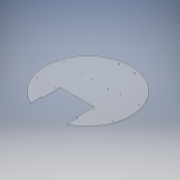
# Autodesk Inventor part: TopPlate
Saved by Autodesk Inventor 2019 (Build 230136000, 136)
## iProperties
Created: 2019-09-28
Part Number: TopPlate
Material: Generic
Document SubType Name: Modeling
Designer: james
Density: 1 g/cm^3
Appearance: Polycarbonate - Clear
Mass: 617.456 g
Surface Area: 2657.72 cm^2
Volume: 617.456 cm^3
Author: james
Autodesk Inventor part; units mm, degrees
ref_plane "YZ Plane" through (0, 0, 0) normal (1, 0, 0) x (0, 1, 0)
ref_plane "XZ Plane" through (0, 0, 0) normal (0, 1, 0) x (-1, 0, 0)
ref_plane "XY Plane" through (0, 0, 0) normal (0, 0, 1) x (1, 0, 0)
sketch "Sketch1" plane through (0, 0, 0) normal (0, 1, 0) x (-1, 0, 0)
  circle A0 centre (0, 0) radius 203.2
  dimension "d0" = 406.4
  constraints: 1 centre point, 1 coincident
  measures "d0" diameter of A0
extrude "Extrusion1" add sketch "Sketch1" along normal blind 4.7625
sketch "Sketch2" plane through (0, 4.7625, 0) normal (0, 1, 0) x (1, 0, 0)
  point P0 (0, 0)
  point P1 (-88.9, 64)
  point P2 (-176.9, 64)
  point P3 (-88.9, -64)
  point P4 (-176.9, -64)
  dimension "d3" = 0
  dimension "d4" = 0
  dimension "d5" = 0
  dimension "d6" = 0
  dimension "d7" = 128
  dimension "d8" = 88
  dimension "d9" = 64
  dimension "d10" = 88.9
  measures "d3" horizontal distance of point (-176.9, -64) point (-176.9, 64)
  measures "d4" horizontal distance of point (-88.9, -64) point (-88.9, 64)
  measures "d5" vertical distance of point (-176.9, -64) point (-88.9, -64)
  measures "d6" vertical distance of point (-176.9, 64) point (-88.9, 64)
  measures "d7" distance of point (-176.9, -64) point (-176.9, 64)
  measures "d8" distance of point (-176.9, -64) point (-88.9, -64)
  measures "d9" vertical distance of point (-88.9, -64) point (0, 0)
  measures "d10" horizontal distance of point (-88.9, 64) point (0, 0)
hole "Hole1" at (-88.9, 4.7625, -64) at (-176.9, 4.7625, -64) at (-88.9, 4.7625, 64) at (-176.9, 4.7625, 64) direction (0, -1, 0) diameter 3.2766 end through all clearance for "Flat Head Machine Screw (82)" size "#4" standard "Ansi Unified Screw Threads"
sketch "Sketch3" plane through (0, 4.7625, 0) normal (0, 1, 0) x (1, 0, 0)
  point P0 (0, 0)
  point P1 (88.9, 64)
  point P2 (176.9, 64)
  point P3 (88.9, -62)
  point P4 (176.9, -62)
  dimension "d18" = 0
  dimension "d19" = 0
  dimension "d20" = 0
  dimension "d21" = 0
  dimension "d22" = 126
  dimension "d23" = 88
  dimension "d24" = 64
  dimension "d25" = 88.9
  measures "d18" horizontal distance of point (176.9, -62) point (176.9, 64)
  measures "d19" vertical distance of point (88.9, 64) point (176.9, 64)
  measures "d20" vertical distance of point (88.9, -62) point (176.9, -62)
  measures "d21" horizontal distance of point (88.9, 64) point (88.9, -62)
  measures "d22" distance of point (176.9, -62) point (176.9, 64)
  measures "d23" distance of point (88.9, -62) point (176.9, -62)
  measures "d24" vertical distance of point (0, 0) point (88.9, 64)
  measures "d25" horizontal distance of point (0, 0) point (88.9, -62)
hole "Hole2" at (88.9, 4.7625, -64) at (176.9, 4.7625, -64) at (88.9, 4.7625, 62) at (176.9, 4.7625, 62) direction (0, -1, 0) diameter 3.2766 end through all clearance for "Flat Head Machine Screw (82)" size "#4" standard "Ansi Unified Screw Threads"
sketch "Sketch4" plane through (0, 4.7625, 0) normal (0, 1, 0) x (1, 0, 0)
  point P0 (0, 0)
  point P1 (-38.1, 184.15)
  point P2 (38.1, 184.15)
  dimension "d33" = 38.1
  dimension "d34" = 0
  dimension "d35" = 76.2
  dimension "d36" = 184.15
  measures "d33" horizontal distance of point (-38.1, 184.15) point (0, 0)
  measures "d34" vertical distance of point (38.1, 184.15) point (-38.1, 184.15)
  measures "d35" distance of point (-38.1, 184.15) point (38.1, 184.15)
  measures "d36" vertical distance of point (0, 0) point (-38.1, 184.15)
hole "Hole3" at (-38.1, 4.7625, -184.15) at (38.1, 4.7625, -184.15) direction (0, -1, 0) diameter 5.1054 end through all clearance for "Flat Head Machine Screw (82)" size "#10" standard "Ansi Unified Screw Threads"
sketch "Sketch5" plane through (0, 4.7625, 0) normal (0, 1, 0) x (1, 0, 0)
  line L0 (-79.375, -50.8) -> (79.375, -50.8)
  line L1 (79.375, -50.8) -> (79.375, -418.3154)
  line L2 (79.375, -418.3154) -> (-79.375, -418.3154)
  line L3 (-79.375, -418.3154) -> (-79.375, -50.8)
  point P0 (0, 0)
  dimension "d44" = 158.75
  dimension "d45" = 79.375
  dimension "d46" = 50.8
  constraints: 8 end point, 2 parallel, 1 horizontal, 1 perpendicular
  measures "d44" distance of L1.end L2.end
  measures "d45" distance from line of L3 point (0, 0)
  measures "d46" distance from line of L0 point (0, 0)
extrude "Extrusion2" cut sketch "Sketch5" against normal blind 25.4
sketch "Sketch6" plane through (0, 4.7625, 0) normal (0, 1, 0) x (1, 0, 0)
  line L0 (-85.725, -133.35) -> (85.725, -133.35)
  line L1 (85.725, -133.35) -> (85.725, -214.7916)
  line L2 (85.725, -214.7916) -> (-85.725, -214.7916)
  line L3 (-85.725, -214.7916) -> (-85.725, -133.35)
  line L4 (-79.375, -50.8) -> (79.375, -50.8) projected
  line L5 (-79.375, -187.0557) -> (-79.375, -50.8) projected
  line L6 (79.375, -50.8) -> (79.375, -187.0557) projected
  point P0 (0, 0)
  dimension "d49" = 82.55
  dimension "d50" = 6.35
  dimension "d51" = 6.35
  constraints: 8 end point, 2 parallel, 1 horizontal, 1 perpendicular
  measures "d49" distance between parallel lines of L0 L4
  measures "d50" distance between parallel lines of L3 L5
  measures "d51" distance between parallel lines of L6 L1
extrude "Extrusion3" cut sketch "Sketch6" against normal blind 25.4 contours L0 L1 L2 L3
sketch "Sketch7" plane through (0, 4.7625, 0) normal (0, 1, 0) x (1, 0, 0)
  circle A0 centre (38.1, 184.15) radius 2.5527 projected
  circle A1 centre (-38.1, 184.15) radius 2.5527 projected
  point P0 (0, 0)
  point P1 (-38.1, 57.15)
  point P2 (38.1, 57.15)
  dimension "d54" = 0
  dimension "d55" = 127
  dimension "d56" = 0
  dimension "d57" = 127
  measures "d54" horizontal distance of point (-38.1, 57.15) A1.centre
  measures "d55" distance of point (-38.1, 57.15) A1.centre
  measures "d56" horizontal distance of A0.centre point (38.1, 57.15)
  measures "d57" distance of A0.centre point (38.1, 57.15)
hole "Hole4" at (-38.1, 4.7625, -57.15) at (38.1, 4.7625, -57.15) direction (0, -1, 0) diameter 4.4958 end through all clearance for "Flat Head Machine Screw (82)" size "#8" standard "Ansi Unified Screw Threads"
body "Solid1"
